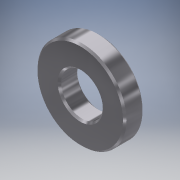
# Autodesk Inventor part: Part33
Saved by Autodesk Inventor 2017.3 (Build 213256000, 256)
## iProperties
Created: 2012-04-09
Part Number: Part33
Material: Steel
Document SubType Name: Modeling
Designer: jhanson2
Density: 7.85 g/cm^3
Appearance: Aluminum - Polished
Mass: 17.0073 g
Surface Area: 13.7219 cm^2
Volume: 2.16653 cm^3
Author: jhanson2
Autodesk Inventor part; units mm, degrees
ref_plane "YZ Plane" through (0, 0, 0) normal (1, 0, 0) x (0, 1, 0)
ref_plane "XZ Plane" through (0, 0, 0) normal (0, 1, 0) x (-1, 0, 0)
ref_plane "XY Plane" through (0, 0, 0) normal (0, 0, 1) x (1, 0, 0)
sketch "Sketch1" plane through (0, 0, 0) normal (0, 0, 1) x (1, 0, 0)
  circle A0 centre (0, 0) radius 5.9531
  circle A1 centre (0, 0) radius 12.7
  dimension "d0" = 11.9062
  dimension "d1" = 25.4
  constraints: 2 centre point, 2 coincident
  measures "d0" diameter of A0
  measures "d1" diameter of A1
extrude "Extrusion1" add sketch "Sketch1" along normal blind 5.5563
chamfer "Chamfer1" distance 0.508 angle 45 4 edges at (-12.7, 0, 5.5563) (-12.7, 0, 0) (-5.9531, 0, 5.5563) (-5.9531, 0, 0)
body "Solid1"
